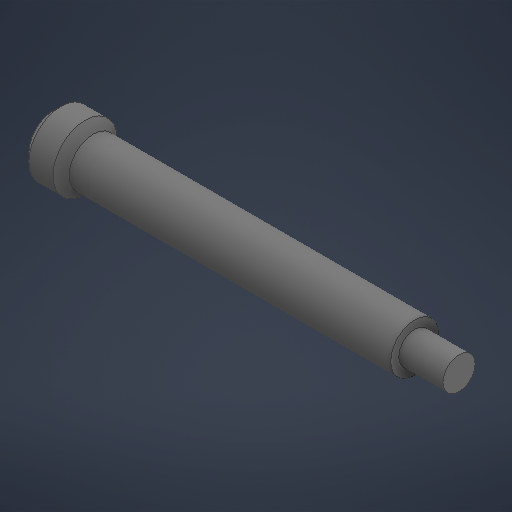
# Autodesk Inventor part: Hajtókar2
Saved by Autodesk Inventor 2025 (Build 290162010, 162A)
## iProperties
Created: 2025-02-13
Part Number: Hajtókar2
Material: Generic
Document SubType Name: Modeling
Designer: petruska.milan
Density: 1 g/cm^3
Appearance: Default
Author: petruska.milan
Autodesk Inventor part; units mm, degrees
ref_plane "YZ Plane" through (0, 0, 0) normal (1, 0, 0) x (0, 1, 0)
ref_plane "XZ Plane" through (0, 0, 0) normal (0, 1, 0) x (-1, 0, 0)
ref_plane "XY Plane" through (0, 0, 0) normal (0, 0, 1) x (1, 0, 0)
sketch "Sketch1" plane through (0, 0, 0) normal (0, 0, 1) x (1, 0, 0)
  line L0 (0, 0) -> (50.5, 0)
  line L1 (50.5, 0) -> (50.5, 3)
  line L2 (50.5, 3) -> (0, 3)
  line L3 (0, 3) -> (0, 0)
  line L4 (0, 0) -> (5, 0)
  line L5 (5, 0) -> (5, 4)
  line L6 (5, 4) -> (0, 4)
  line L7 (0, 4) -> (0, 0)
  line L8 (50.5, 0) -> (45, 0)
  line L9 (45, 0) -> (45, 2)
  line L10 (45, 2) -> (50.5, 2)
  line L11 (50.5, 2) -> (50.5, 0)
  line L12 (45, 2) -> (45, 3)
  point P0 (5, 3)
  dimension "d0" = 50.5
  dimension "d1" = 3
  dimension "d2" = 5
  dimension "d3" = 4
  dimension "d4" = 5.5
  dimension "d5" = 2
  constraints: 26 end point, 6 parallel, 4 perpendicular, 3 horizontal, 1 point on line
  measures "d0" distance of L2.end L1.end
  measures "d1" distance of L1.end L0.end
  measures "d2" distance of L6.end L5.end
  measures "d3" distance of L5.end L4.end
  measures "d4" distance of L9.end L10.end
  measures "d5" distance of L8.end L9.end
revolve "Revolution1" add sketch "Sketch1" angle 360 about axis through (0, 0, 0) along (1, 0, 0) contours L3 L2 L5 L0 | L5 L2 L12 L9 L0 | L7 L6 L5 L2 | L9 L10 L1 L0
chamfer "Chamfer1" distance 1 angle 45 2 edges at (5, -4, 0) (0, -4, 0)
body "Solid1"
